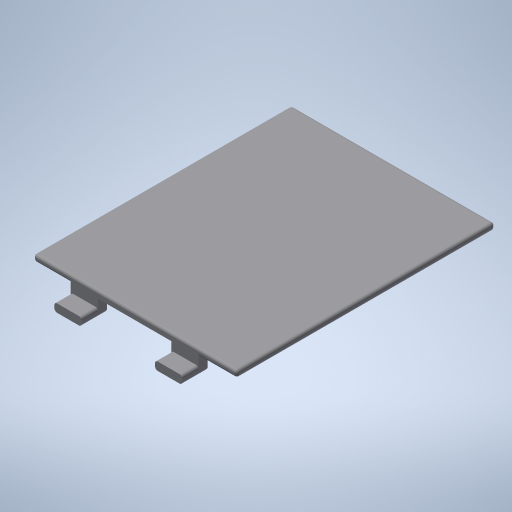
# Autodesk Inventor part: tapa decaja 2
Saved by Autodesk Inventor 2023 (Build 270158000, 158)
## iProperties
Created: 2022-11-17
Part Number: tapa decaja 2
Material: Generic
Document SubType Name: Modeling
Designer: Xiaba
Density: 1 g/cm^3
Appearance: Default
Author: Xiaba
Autodesk Inventor part; units mm, degrees
ref_plane "YZ Plane" through (0, 0, 0) normal (1, 0, 0) x (0, 1, 0)
ref_plane "XZ Plane" through (0, 0, 0) normal (0, 1, 0) x (-1, 0, 0)
ref_plane "XY Plane" through (0, 0, 0) normal (0, 0, 1) x (1, 0, 0)
sketch "Sketch1" plane through (0, 0, 0) normal (0, 1, 0) x (-1, 0, 0)
  line L0 (36.4, 47.4) -> (-36.4, 47.4)
  line L1 (-37.4, 46.4) -> (-37.4, -46.4)
  line L2 (-36.4, -47.4) -> (36.4, -47.4)
  line L3 (37.4, -46.4) -> (37.4, 46.4)
  line L4 (37.4, 47.4) -> (-37.4, -47.4) construction
  line L5 (-37.4, 47.4) -> (37.4, -47.4) construction
  arc A0 (37.4, 46.4) -> (36.4, 47.4) centre (36.4, 46.4) ccw
  arc A1 (-36.4, 47.4) -> (-37.4, 46.4) centre (-36.4, 46.4) ccw
  arc A2 (-37.4, -46.4) -> (-36.4, -47.4) centre (-36.4, -46.4) ccw
  arc A3 (36.4, -47.4) -> (37.4, -46.4) centre (36.4, -46.4) ccw
  point P0 (0, 0)
  dimension "d0" = 94.8
  dimension "d1" = 74.8
  dimension "d2" = 1
  constraints: 12 end point, 8 point on circle, 8 point on line, 8 tangent, 4 centre point, 3 equal radius, 2 midpoint, 2 parallel, 1 horizontal, 1 perpendicular
  measures "d0" distance of L5.end L4.start
  measures "d1" distance of L4.end L5.end
  measures "d2" radius of A0
extrude "Extrusion1" add sketch "Sketch1" along normal blind 2.5
sketch "Sketch2" plane through (0, 0, 0) normal (0, -1, 0) x (1, 0, 0)
  line L0 (0, 0) -> (-37.4, 0)
  line L1 (-37.4, 0) -> (-37.4, 47.4)
  line L2 (-37.4, 47.4) -> (0, 47.4)
  line L3 (0, 47.4) -> (0, 0)
  line L4 (-23.7, 51.4) -> (-13.7, 51.4)
  line L5 (-13.7, 51.4) -> (-13.7, 43.4)
  line L6 (-13.7, 43.4) -> (-23.7, 43.4)
  line L7 (-23.7, 43.4) -> (-23.7, 51.4)
  line L8 (-36.4, 47.4) -> (36.4, 47.4) projected
  line L9 (-23.7, 51.4) -> (-13.7, 43.4) construction
  line L10 (-13.7, 51.4) -> (-23.7, 43.4) construction
  line L11 (0, 0) -> (36.5961, 0)
  line L12 (36.5961, 0) -> (36.5961, 47.4)
  line L13 (36.5961, 47.4) -> (0, 47.4)
  line L14 (0, 47.4) -> (0, 0)
  line L15 (13.2981, 51.4) -> (23.2981, 51.4)
  line L16 (23.2981, 51.4) -> (23.2981, 43.4)
  line L17 (23.2981, 43.4) -> (13.2981, 43.4)
  line L18 (13.2981, 43.4) -> (13.2981, 51.4)
  line L19 (13.2981, 51.4) -> (23.2981, 43.4) construction
  line L20 (23.2981, 51.4) -> (13.2981, 43.4) construction
  point P0 (-18.7, 47.4)
  point P1 (18.2981, 47.4)
  point P2 (23.2981, 47.4)
  point P3 (13.2981, 47.4)
  point P4 (-13.7, 47.4)
  point P5 (-23.7, 47.4)
  dimension "d5" = 10
  dimension "d6" = 8
  dimension "d7" = 10
  dimension "d8" = 8
  constraints: 40 end point, 8 parallel, 5 midpoint, 4 horizontal, 4 perpendicular, 1 point on line
  measures "d5" distance of L4.start L4.end
  measures "d6" distance of L4.end L5.end
  measures "d7" distance of L15.start L15.end
  measures "d8" distance of L15.end L16.end
extrude "Extrusion2" add sketch "Sketch2" along normal blind 6 contours L5 L6 L7 L2 | L8 L16 L17 L18
sketch "Sketch3" plane through (-36.4, 2.5, 47.4) normal (0, 0, 1) x (1, 0, 0)
  line L0 (12.7, -8.5) -> (22.7, -8.5) projected
  line L1 (22.7, -2.5) -> (22.7, -8.5) projected
  line L2 (13.7, -8.5) -> (21.7, -8.5)
  line L3 (22.7, -7.5) -> (22.7, -6.5)
  line L4 (21.7, -5.5) -> (13.7, -5.5)
  line L5 (12.7, -6.5) -> (12.7, -7.5)
  line L6 (59.6981, -2.5) -> (59.6981, -8.5) projected
  line L7 (50.6981, -8.5) -> (58.6981, -8.5)
  line L8 (59.6981, -7.5) -> (59.6981, -6.5)
  line L9 (58.6981, -5.5) -> (50.6981, -5.5)
  line L10 (49.6981, -6.5) -> (49.6981, -7.5)
  arc A0 (13.7, -5.5) -> (12.7, -6.5) centre (13.7, -6.5) ccw
  arc A1 (22.7, -6.5) -> (21.7, -5.5) centre (21.7, -6.5) ccw
  arc A2 (21.7, -8.5) -> (22.7, -7.5) centre (21.7, -7.5) ccw
  arc A3 (12.7, -7.5) -> (13.7, -8.5) centre (13.7, -7.5) ccw
  arc A4 (50.6981, -5.5) -> (49.6981, -6.5) centre (50.6981, -6.5) ccw
  arc A5 (59.6981, -6.5) -> (58.6981, -5.5) centre (58.6981, -6.5) ccw
  arc A6 (58.6981, -8.5) -> (59.6981, -7.5) centre (58.6981, -7.5) ccw
  arc A7 (49.6981, -7.5) -> (50.6981, -8.5) centre (50.6981, -7.5) ccw
  line L11 (49.0159, -7.1882) -> (60.5232, -7.1882)
  line L12 (60.5232, -7.1882) -> (60.5232, -9.9786)
  line L13 (60.5232, -9.9786) -> (49.0159, -9.9786)
  line L14 (49.0159, -9.9786) -> (49.0159, -7.1882)
  line L15 (11.7436, -7.1882) -> (24.9599, -7.1882)
  line L16 (24.9599, -7.1882) -> (24.9599, -11.0237)
  line L17 (24.9599, -11.0237) -> (11.7436, -11.0237)
  line L18 (11.7436, -11.0237) -> (11.7436, -7.1882)
  line L19 (49.6981, -8.5) -> (59.6981, -8.5) projected
  line L20 (49.0159, -8.5834) -> (59.6981, -8.5)
  line L21 (49.6981, -8.5) -> (59.6981, -8.5)
  point P0 (36.4, -2.5)
  point P1 (22.7, -5.5)
  point P2 (59.6981, -5.5)
  point P3 (12.7, -7.1882)
  point P4 (22.7, -7.1882)
  point P5 (49.6981, -7.1882)
  dimension "d11" = 1
  constraints: 36 end point, 16 point on circle, 16 tangent, 9 point on line, 8 centre point, 8 parallel, 7 equal radius, 5 horizontal, 4 perpendicular, 3 midpoint
  measures "d11" radius of A0
extrude "Extrusion3" add sketch "Sketch3" along normal blind 6 contours A3 L5 L15 L1 A2 L0 | L5 A0 L4 A1 L1 L15 | A6 L7 A7 L10 L11 L6 | L11 L10 A4 L9 A5 L6
extrude "Extrusion4" cut sketch "Sketch3" against normal blind 6 contours L0 L1 L15 L16 L17 L18 L5 A3 | A2 L1 L0 | L6 L19 A6 | L20 L14 L11 L10 A7 L7 L19
fillet "Fillet1" radius 1 10 edges at (23.0052, -5.7071, 43.4) (18.2981, -6, 43.4) (13.591, -5.7071, 43.4) (13.2981, -2.5, 43.4) (23.2981, -2.5, 43.4) (-13.9929, -5.7071, 43.4) (-18.7, -6, 43.4) (-23.4071, -5.7071, 43.4) (-23.7, -2.5, 43.4) (-13.7, -2.5, 43.4)
fillet "Fillet2" radius 1 17 edges at (37.1071, 0, -47.1071) (0, 0, -47.4) (-37.1071, 0, -47.1071) (-37.4, 0, 0) (-37.1071, 0, 47.1071) (-30.05, 0, 47.4) (37.1071, 0, 47.1071) (29.849, 0, 47.4) (37.4, 0, 0) (37.1071, 2.5, -47.1071) (0, 2.5, -47.4) (-37.1071, 2.5, -47.1071) (-37.4, 2.5, 0) (-37.1071, 2.5, 47.1071) (0, 2.5, 47.4) (37.1071, 2.5, 47.1071) (37.4, 2.5, 0)
body "Solid1"
